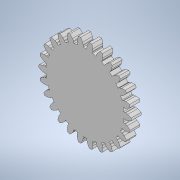
# Autodesk Inventor part: m1歯数26ギア3t
Saved by Autodesk Inventor 2020.2 (Build 242310000, 310)
## iProperties
Created: 2020-02-29
Part Number: m1歯数26ギア3t
Material: 一般
Document SubType Name: Modeling
Designer: aoyam
Density: 1 g/cm^3
Appearance: 既定
Author: aoyam
Autodesk Inventor part; units mm, degrees
ref_plane "YZ Plane" through (0, 0, 0) normal (1, 0, 0) x (0, 1, 0)
ref_plane "XZ Plane" through (0, 0, 0) normal (0, 1, 0) x (-1, 0, 0)
ref_plane "XY Plane" through (0, 0, 0) normal (0, 0, 1) x (1, 0, 0)
sketch "スケッチ1" plane through (0, 0, 0) normal (0, 0, 1) x (1, 0, 0)
  arc A0 (2.4708, 13.787) -> (2.4421, 13.6092) centre (3.6157, 13.511) ccw
  arc A1 (2.6541, 14.342) -> (2.4708, 13.787) centre (5.6233, 13.0538) ccw
  arc A2 (3.2141, 15.3428) -> (2.6541, 14.342) centre (7.7861, 12.1274) ccw
  arc A3 (1.3306, 13.6092) -> (1.3019, 13.787) centre (0.157, 13.511) ccw
  arc A4 (1.3019, 13.787) -> (1.1186, 14.342) centre (-1.8506, 13.0538) ccw
  arc A5 (1.1186, 14.342) -> (0.5586, 15.3428) centre (-4.0134, 12.1274) ccw
  arc A6 (2.4209, 13.1437) -> (1.3518, 13.1437) centre (1.8864, 1.4059) ccw
  arc A7 (0.5586, 15.3428) -> (-0.1598, 15.2555) centre (1.8864, 1.4059) ccw
  line L0 (2.4209, 13.1437) -> (2.4421, 13.6092)
  line L1 (1.3518, 13.1437) -> (1.3306, 13.6092)
  arc A8 (-0.5092, 13.5671) -> (-0.4945, 13.3876) centre (0.6685, 13.5731) ccw
  arc A9 (-1.6441, 13.2874) -> (-1.9549, 13.7824) centre (-4.5296, 11.821) ccw
  arc A10 (-0.1598, 15.2555) -> (-0.464, 14.1498) centre (5.0489, 13.2277) ccw
  arc A11 (-1.9549, 13.7824) -> (-2.7381, 14.6201) centre (-6.4078, 10.4039) ccw
  arc A12 (-2.7381, 14.6201) -> (-3.4148, 14.3634) centre (1.8864, 1.4059) ccw
  arc A13 (-1.5737, 13.1216) -> (-1.6441, 13.2874) centre (-2.6897, 12.7454) ccw
  line L2 (-1.4417, 12.6747) -> (-1.5737, 13.1216)
  arc A14 (-0.4037, 12.9306) -> (-1.4417, 12.6747) centre (1.8864, 1.4059) ccw
  line L3 (-0.4037, 12.9306) -> (-0.4945, 13.3876)
  arc A15 (-0.464, 14.1498) -> (-0.5092, 13.5671) centre (2.7272, 13.6096) ccw
  arc A16 (-3.3499, 12.6405) -> (-3.2927, 12.4697) centre (-2.2079, 12.9281) ccw
  arc A17 (-4.385, 12.0972) -> (-4.8051, 12.5035) centre (-6.8356, 9.9829) ccw
  arc A18 (-3.4148, 14.3634) -> (-3.4456, 13.217) centre (2.1278, 13.641) ccw
  arc A19 (-4.8051, 12.5035) -> (-5.7661, 13.1294) centre (-8.3201, 8.1575) ccw
  arc A20 (-5.7661, 13.1294) -> (-6.3617, 12.7182) centre (1.8864, 1.4059) ccw
  arc A21 (-4.2769, 11.9531) -> (-4.385, 12.0972) centre (-5.2705, 11.3208) ccw
  line L4 (-4.0418, 11.5508) -> (-4.2769, 11.9531)
  arc A22 (-3.0951, 12.0476) -> (-4.0418, 11.5508) centre (1.8864, 1.4059) ccw
  line L5 (-3.0951, 12.0476) -> (-3.2927, 12.4697)
  arc A23 (-3.4456, 13.217) -> (-3.3499, 12.6405) centre (-0.2178, 13.4562) ccw
  arc A24 (-5.8864, 11.0609) -> (-5.79, 10.9088) centre (-4.8464, 11.6135) ccw
  arc A25 (-6.7613, 10.2857) -> (-7.2665, 10.5796) centre (-8.6348, 7.6464) ccw
  arc A26 (-6.3617, 12.7182) -> (-6.1172, 11.5978) centre (-0.8073, 13.3433) ccw
  arc A27 (-7.2665, 10.5796) -> (-8.3493, 10.9574) centre (-9.6393, 5.5188) ccw
  arc A28 (-8.3493, 10.9574) -> (-8.8293, 10.4156) centre (1.8864, 1.4059) ccw
  arc A29 (-6.622, 10.1717) -> (-6.7613, 10.2857) centre (-7.4353, 9.3199) ccw
  line L6 (-6.2974, 9.8373) -> (-6.622, 10.1717)
  arc A30 (-5.4971, 10.5463) -> (-6.2974, 9.8373) centre (1.8864, 1.4059) ccw
  line L7 (-5.4971, 10.5463) -> (-5.79, 10.9088)
  arc A31 (-6.1172, 11.5978) -> (-5.8864, 11.0609) centre (-3.0405, 12.6025) ccw
  arc A32 (-7.9711, 8.9202) -> (-7.8411, 8.7956) centre (-7.0936, 9.7056) ccw
  arc A33 (-8.6351, 7.9582) -> (-9.196, 8.1226) centre (-9.8225, 4.9472) ccw
  arc A34 (-8.8293, 10.4156) -> (-8.3237, 9.3862) centre (-3.5858, 12.3518) ccw
  arc A35 (-9.196, 8.1226) -> (-10.3377, 8.2302) centre (-10.2887, 2.641) ccw
  arc A36 (-10.3377, 8.2302) -> (-10.6741, 7.5894) centre (1.8864, 1.4059) ccw
  arc A37 (-8.4725, 7.8808) -> (-8.6351, 7.9582) centre (-9.0584, 6.8591) ccw
  line L8 (-8.0774, 7.6338) -> (-8.4725, 7.8808)
  arc A38 (-7.47, 8.5137) -> (-8.0774, 7.6338) centre (1.8864, 1.4059) ccw
  line L9 (-7.47, 8.5137) -> (-7.8411, 8.7956)
  arc A39 (-8.3237, 9.3862) -> (-7.9711, 8.9202) centre (-5.5768, 11.0981) ccw
  arc A40 (-9.483, 6.3428) -> (-9.3269, 6.2529) centre (-8.8189, 7.3154) ccw
  arc A41 (-9.8975, 5.2498) -> (-10.4813, 5.2753) centre (-10.3298, 2.0422) ccw
  arc A42 (-10.6741, 7.5894) -> (-9.9369, 6.7109) centre (-6.0463, 10.7241) ccw
  arc A43 (-10.4813, 5.2753) -> (-11.6157, 5.1065) centre (-10.2305, -0.3086) ccw
  arc A44 (-11.6157, 5.1065) -> (-11.7889, 4.4038) centre (1.8864, 1.4059) ccw
  arc A45 (-9.7211, 5.2136) -> (-9.8975, 5.2498) centre (-10.0454, 4.0814) ccw
  line L10 (-9.2783, 5.0683) -> (-9.7211, 5.2136)
  arc A46 (-8.8991, 6.068) -> (-9.2783, 5.0683) centre (1.8864, 1.4059) ccw
  line L11 (-8.8991, 6.068) -> (-9.3269, 6.2529)
  arc A47 (-9.9369, 6.7109) -> (-9.483, 6.3428) centre (-7.6795, 9.0304) ccw
  arc A48 (-10.3341, 3.4785) -> (-10.161, 3.4286) centre (-9.9221, 4.5818) ccw
  arc A49 (-10.475, 2.3181) -> (-11.048, 2.203) centre (-10.1271, -0.8998) ccw
  arc A50 (-11.7889, 4.4038) -> (-10.8629, 3.7273) centre (-8.0458, 8.555) ccw
  arc A51 (-11.048, 2.203) -> (-12.109, 1.7677) centre (-9.4681, -3.1585) ccw
  arc A52 (-12.109, 1.7677) -> (-12.109, 1.044) centre (1.8864, 1.4059) ccw
  arc A53 (-10.295, 2.3251) -> (-10.475, 2.3181) centre (-10.339, 1.1482) ccw
  line L12 (-9.8303, 2.2901) -> (-10.295, 2.3251)
  arc A54 (-9.7015, 3.3514) -> (-9.8303, 2.2901) centre (1.8864, 1.4059) ccw
  line L13 (-9.7015, 3.3514) -> (-10.161, 3.4286)
  arc A55 (-10.8629, 3.7273) -> (-10.3341, 3.4785) centre (-9.2262, 6.5196) ccw
  arc A56 (-10.475, 0.4937) -> (-10.295, 0.4866) centre (-10.339, 1.6635) ccw
  arc A57 (-10.3341, -0.6667) -> (-10.8629, -0.9155) centre (-9.2262, -3.7078) ccw
  arc A58 (-12.109, 1.044) -> (-11.048, 0.6087) centre (-9.4681, 5.9703) ccw
  arc A59 (-10.8629, -0.9155) -> (-11.7889, -1.5921) centre (-8.0458, -5.7432) ccw
  arc A60 (-11.7889, -1.5921) -> (-11.6157, -2.2948) centre (1.8864, 1.4059) ccw
  arc A61 (-10.161, -0.6168) -> (-10.3341, -0.6667) centre (-9.9221, -1.77) ccw
  line L14 (-9.7015, -0.5396) -> (-10.161, -0.6168)
  arc A62 (-9.8303, 0.5217) -> (-9.7015, -0.5396) centre (1.8864, 1.4059) ccw
  line L15 (-9.8303, 0.5217) -> (-10.295, 0.4866)
  arc A63 (-11.048, 0.6087) -> (-10.475, 0.4937) centre (-10.1271, 3.7116) ccw
  arc A64 (-9.8975, -2.438) -> (-9.7211, -2.4018) centre (-10.0454, -1.2697) ccw
  arc A65 (-9.483, -3.531) -> (-9.9369, -3.8991) centre (-7.6795, -6.2186) ccw
  arc A66 (-11.6157, -2.2948) -> (-10.4813, -2.4635) centre (-10.2305, 3.1204) ccw
  arc A67 (-9.9369, -3.8991) -> (-10.6741, -4.7777) centre (-6.0463, -7.9124) ccw
  arc A68 (-10.6741, -4.7777) -> (-10.3377, -5.4185) centre (1.8864, 1.4059) ccw
  arc A69 (-9.3269, -3.4411) -> (-9.483, -3.531) centre (-8.8189, -4.5036) ccw
  line L16 (-8.8991, -3.2562) -> (-9.3269, -3.4411)
  arc A70 (-9.2783, -2.2566) -> (-8.8991, -3.2562) centre (1.8864, 1.4059) ccw
  line L17 (-9.2783, -2.2566) -> (-9.7211, -2.4018)
  arc A71 (-10.4813, -2.4635) -> (-9.8975, -2.438) centre (-10.3298, 0.7696) ccw
  arc A72 (-8.6351, -5.1464) -> (-8.4725, -5.069) centre (-9.0584, -4.0474) ccw
  arc A73 (-7.9711, -6.1084) -> (-8.3237, -6.5745) centre (-5.5768, -8.2863) ccw
  arc A74 (-10.3377, -5.4185) -> (-9.196, -5.3108) centre (-10.2887, 0.1708) ccw
  arc A75 (-8.3237, -6.5745) -> (-8.8293, -7.6039) centre (-3.5858, -9.54) ccw
  arc A76 (-8.8293, -7.6039) -> (-8.3493, -8.1456) centre (1.8864, 1.4059) ccw
  arc A77 (-7.8411, -5.9838) -> (-7.9711, -6.1084) centre (-7.0936, -6.8939) ccw
  line L18 (-7.47, -5.7019) -> (-7.8411, -5.9838)
  arc A78 (-8.0774, -4.822) -> (-7.47, -5.7019) centre (1.8864, 1.4059) ccw
  line L19 (-8.0774, -4.822) -> (-8.4725, -5.069)
  arc A79 (-9.196, -5.3108) -> (-8.6351, -5.1464) centre (-9.8225, -2.1354) ccw
  arc A80 (-6.7613, -7.474) -> (-6.622, -7.3599) centre (-7.4353, -6.5082) ccw
  arc A81 (-5.8864, -8.2491) -> (-6.1172, -8.786) centre (-3.0405, -9.7908) ccw
  arc A82 (-8.3493, -8.1456) -> (-7.2665, -7.7678) centre (-9.6393, -2.707) ccw
  arc A83 (-6.1172, -8.786) -> (-6.3617, -9.9065) centre (-0.8073, -10.5315) ccw
  arc A84 (-6.3617, -9.9065) -> (-5.7661, -10.3176) centre (1.8864, 1.4059) ccw
  arc A85 (-5.79, -8.097) -> (-5.8864, -8.2491) centre (-4.8464, -8.8017) ccw
  line L20 (-5.4971, -7.7345) -> (-5.79, -8.097)
  arc A86 (-6.2974, -7.0255) -> (-5.4971, -7.7345) centre (1.8864, 1.4059) ccw
  line L21 (-6.2974, -7.0255) -> (-6.622, -7.3599)
  arc A87 (-7.2665, -7.7678) -> (-6.7613, -7.474) centre (-8.6348, -4.8346) ccw
  arc A88 (-4.385, -9.2855) -> (-4.2769, -9.1414) centre (-5.2705, -8.509) ccw
  arc A89 (-3.3499, -9.8287) -> (-3.4456, -10.4052) centre (-0.2178, -10.6445) ccw
  arc A90 (-5.7661, -10.3176) -> (-4.8051, -9.6917) centre (-8.3201, -5.3458) ccw
  arc A91 (-3.4456, -10.4052) -> (-3.4148, -11.5517) centre (2.1278, -10.8293) ccw
  arc A92 (-3.4148, -11.5517) -> (-2.7381, -11.8083) centre (1.8864, 1.4059) ccw
  arc A93 (-3.2927, -9.6579) -> (-3.3499, -9.8287) centre (-2.2079, -10.1163) ccw
  line L22 (-3.0951, -9.2359) -> (-3.2927, -9.6579)
  arc A94 (-4.0418, -8.739) -> (-3.0951, -9.2359) centre (1.8864, 1.4059) ccw
  line L23 (-4.0418, -8.739) -> (-4.2769, -9.1414)
  arc A95 (-4.8051, -9.6917) -> (-4.385, -9.2855) centre (-6.8356, -7.1712) ccw
  arc A96 (-1.6441, -10.4756) -> (-1.5737, -10.3099) centre (-2.6897, -9.9336) ccw
  arc A97 (-0.5092, -10.7554) -> (-0.464, -11.338) centre (2.7272, -10.7979) ccw
  arc A98 (-2.7381, -11.8083) -> (-1.9549, -10.9706) centre (-6.4078, -7.5922) ccw
  arc A99 (-0.464, -11.338) -> (-0.1598, -12.4438) centre (5.0489, -10.416) ccw
  arc A100 (-0.1598, -12.4438) -> (0.5586, -12.531) centre (1.8864, 1.4059) ccw
  arc A101 (-0.4945, -10.5759) -> (-0.5092, -10.7554) centre (0.6685, -10.7614) ccw
  line L24 (-0.4037, -10.1188) -> (-0.4945, -10.5759)
  arc A102 (-1.4417, -9.8629) -> (-0.4037, -10.1188) centre (1.8864, 1.4059) ccw
  line L25 (-1.4417, -9.8629) -> (-1.5737, -10.3099)
  arc A103 (-1.9549, -10.9706) -> (-1.6441, -10.4756) centre (-4.5296, -9.0092) ccw
  arc A104 (1.3019, -10.9753) -> (1.3306, -10.7975) centre (0.157, -10.6992) ccw
  arc A105 (2.4708, -10.9753) -> (2.6541, -11.5302) centre (5.6233, -10.242) ccw
  arc A106 (0.5586, -12.531) -> (1.1186, -11.5302) centre (-4.0134, -9.3156) ccw
  arc A107 (2.6541, -11.5302) -> (3.2141, -12.531) centre (7.7861, -9.3156) ccw
  arc A108 (3.2141, -12.531) -> (3.9325, -12.4438) centre (1.8864, 1.4059) ccw
  arc A109 (2.4421, -10.7975) -> (2.4708, -10.9753) centre (3.6157, -10.6992) ccw
  line L26 (2.4209, -10.3319) -> (2.4421, -10.7975)
  arc A110 (1.3518, -10.3319) -> (2.4209, -10.3319) centre (1.8864, 1.4059) ccw
  line L27 (1.3518, -10.3319) -> (1.3306, -10.7975)
  arc A111 (1.1186, -11.5302) -> (1.3019, -10.9753) centre (-1.8506, -10.242) ccw
  arc A112 (4.2819, -10.7554) -> (4.2672, -10.5759) centre (3.1042, -10.7614) ccw
  arc A113 (5.4168, -10.4756) -> (5.7276, -10.9706) centre (8.3023, -9.0092) ccw
  arc A114 (3.9325, -12.4438) -> (4.2368, -11.338) centre (-1.2761, -10.416) ccw
  arc A115 (5.7276, -10.9706) -> (6.5108, -11.8083) centre (10.1805, -7.5922) ccw
  arc A116 (6.5108, -11.8083) -> (7.1875, -11.5517) centre (1.8864, 1.4059) ccw
  arc A117 (5.3464, -10.3099) -> (5.4168, -10.4756) centre (6.4624, -9.9336) ccw
  line L28 (5.2144, -9.8629) -> (5.3464, -10.3099)
  arc A118 (4.1764, -10.1188) -> (5.2144, -9.8629) centre (1.8864, 1.4059) ccw
  line L29 (4.1764, -10.1188) -> (4.2672, -10.5759)
  arc A119 (4.2368, -11.338) -> (4.2819, -10.7554) centre (1.0455, -10.7979) ccw
  arc A120 (7.1226, -9.8287) -> (7.0654, -9.6579) centre (5.9806, -10.1163) ccw
  arc A121 (8.1577, -9.2855) -> (8.5778, -9.6917) centre (10.6083, -7.1712) ccw
  arc A122 (7.1875, -11.5517) -> (7.2183, -10.4052) centre (1.6449, -10.8293) ccw
  arc A123 (8.5778, -9.6917) -> (9.5388, -10.3176) centre (12.0928, -5.3458) ccw
  arc A124 (9.5388, -10.3176) -> (10.1344, -9.9065) centre (1.8864, 1.4059) ccw
  arc A125 (8.0496, -9.1414) -> (8.1577, -9.2855) centre (9.0432, -8.509) ccw
  line L30 (7.8145, -8.739) -> (8.0496, -9.1414)
  arc A126 (6.8679, -9.2359) -> (7.8145, -8.739) centre (1.8864, 1.4059) ccw
  line L31 (6.8679, -9.2359) -> (7.0654, -9.6579)
  arc A127 (7.2183, -10.4052) -> (7.1226, -9.8287) centre (3.9905, -10.6445) ccw
  arc A128 (9.6591, -8.2491) -> (9.5627, -8.097) centre (8.6191, -8.8017) ccw
  arc A129 (10.5341, -7.474) -> (11.0392, -7.7678) centre (12.4075, -4.8346) ccw
  arc A130 (10.1344, -9.9065) -> (9.8899, -8.786) centre (4.58, -10.5315) ccw
  arc A131 (11.0392, -7.7678) -> (12.122, -8.1456) centre (13.412, -2.707) ccw
  arc A132 (12.122, -8.1456) -> (12.602, -7.6039) centre (1.8864, 1.4059) ccw
  arc A133 (10.3947, -7.3599) -> (10.5341, -7.474) centre (11.208, -6.5082) ccw
  line L32 (10.0701, -7.0255) -> (10.3947, -7.3599)
  arc A134 (9.2699, -7.7345) -> (10.0701, -7.0255) centre (1.8864, 1.4059) ccw
  line L33 (9.2699, -7.7345) -> (9.5627, -8.097)
  arc A135 (9.8899, -8.786) -> (9.6591, -8.2491) centre (6.8132, -9.7908) ccw
  arc A136 (11.7438, -6.1084) -> (11.6138, -5.9838) centre (10.8663, -6.8939) ccw
  arc A137 (12.4079, -5.1464) -> (12.9687, -5.3108) centre (13.5952, -2.1354) ccw
  arc A138 (12.602, -7.6039) -> (12.0964, -6.5745) centre (7.3585, -9.54) ccw
  arc A139 (12.9687, -5.3108) -> (14.1104, -5.4185) centre (14.0614, 0.1708) ccw
  arc A140 (14.1104, -5.4185) -> (14.4468, -4.7777) centre (1.8864, 1.4059) ccw
  arc A141 (12.2452, -5.069) -> (12.4079, -5.1464) centre (12.8311, -4.0474) ccw
  line L34 (11.8501, -4.822) -> (12.2452, -5.069)
  arc A142 (11.2427, -5.7019) -> (11.8501, -4.822) centre (1.8864, 1.4059) ccw
  line L35 (11.2427, -5.7019) -> (11.6138, -5.9838)
  arc A143 (12.0964, -6.5745) -> (11.7438, -6.1084) centre (9.3495, -8.2863) ccw
  arc A144 (13.2557, -3.531) -> (13.0996, -3.4411) centre (12.5916, -4.5036) ccw
  arc A145 (13.6702, -2.438) -> (14.2541, -2.4635) centre (14.1025, 0.7696) ccw
  arc A146 (14.4468, -4.7777) -> (13.7096, -3.8991) centre (9.819, -7.9124) ccw
  arc A147 (14.2541, -2.4635) -> (15.3884, -2.2948) centre (14.0032, 3.1204) ccw
  arc A148 (15.3884, -2.2948) -> (15.5616, -1.5921) centre (1.8864, 1.4059) ccw
  arc A149 (13.4938, -2.4018) -> (13.6702, -2.438) centre (13.8181, -1.2697) ccw
  line L36 (13.051, -2.2566) -> (13.4938, -2.4018)
  arc A150 (12.6719, -3.2562) -> (13.051, -2.2566) centre (1.8864, 1.4059) ccw
  line L37 (12.6719, -3.2562) -> (13.0996, -3.4411)
  arc A151 (13.7096, -3.8991) -> (13.2557, -3.531) centre (11.4522, -6.2186) ccw
  arc A152 (14.1068, -0.6667) -> (13.9337, -0.6168) centre (13.6948, -1.77) ccw
  arc A153 (14.2477, 0.4937) -> (14.8207, 0.6087) centre (13.8998, 3.7116) ccw
  arc A154 (15.5616, -1.5921) -> (14.6356, -0.9155) centre (11.8185, -5.7432) ccw
  arc A155 (14.8207, 0.6087) -> (15.8817, 1.044) centre (13.2408, 5.9703) ccw
  arc A156 (15.8817, 1.044) -> (15.8817, 1.7677) centre (1.8864, 1.4059) ccw
  arc A157 (14.0677, 0.4866) -> (14.2477, 0.4937) centre (14.1117, 1.6635) ccw
  line L38 (13.603, 0.5217) -> (14.0677, 0.4866)
  arc A158 (13.4742, -0.5396) -> (13.603, 0.5217) centre (1.8864, 1.4059) ccw
  line L39 (13.4742, -0.5396) -> (13.9337, -0.6168)
  arc A159 (14.6356, -0.9155) -> (14.1068, -0.6667) centre (12.9989, -3.7078) ccw
  arc A160 (14.2477, 2.3181) -> (14.0677, 2.3251) centre (14.1117, 1.1482) ccw
  arc A161 (14.1068, 3.4785) -> (14.6356, 3.7273) centre (12.9989, 6.5196) ccw
  arc A162 (15.8817, 1.7677) -> (14.8207, 2.203) centre (13.2408, -3.1585) ccw
  arc A163 (14.6356, 3.7273) -> (15.5616, 4.4038) centre (11.8185, 8.555) ccw
  arc A164 (15.5616, 4.4038) -> (15.3884, 5.1065) centre (1.8864, 1.4059) ccw
  arc A165 (13.9337, 3.4286) -> (14.1068, 3.4785) centre (13.6948, 4.5818) ccw
  line L40 (13.4742, 3.3514) -> (13.9337, 3.4286)
  arc A166 (13.603, 2.2901) -> (13.4742, 3.3514) centre (1.8864, 1.4059) ccw
  line L41 (13.603, 2.2901) -> (14.0677, 2.3251)
  arc A167 (14.8207, 2.203) -> (14.2477, 2.3181) centre (13.8998, -0.8998) ccw
  arc A168 (13.6702, 5.2498) -> (13.4938, 5.2136) centre (13.8181, 4.0814) ccw
  arc A169 (13.2557, 6.3428) -> (13.7096, 6.7109) centre (11.4522, 9.0304) ccw
  arc A170 (15.3884, 5.1065) -> (14.2541, 5.2753) centre (14.0032, -0.3086) ccw
  arc A171 (13.7096, 6.7109) -> (14.4468, 7.5894) centre (9.819, 10.7241) ccw
  arc A172 (14.4468, 7.5894) -> (14.1104, 8.2302) centre (1.8864, 1.4059) ccw
  arc A173 (13.0996, 6.2529) -> (13.2557, 6.3428) centre (12.5916, 7.3154) ccw
  line L42 (12.6719, 6.068) -> (13.0996, 6.2529)
  arc A174 (13.051, 5.0683) -> (12.6719, 6.068) centre (1.8864, 1.4059) ccw
  line L43 (13.051, 5.0683) -> (13.4938, 5.2136)
  arc A175 (14.2541, 5.2753) -> (13.6702, 5.2498) centre (14.1025, 2.0422) ccw
  arc A176 (12.4079, 7.9582) -> (12.2452, 7.8808) centre (12.8311, 6.8591) ccw
  arc A177 (11.7438, 8.9202) -> (12.0964, 9.3862) centre (9.3495, 11.0981) ccw
  arc A178 (14.1104, 8.2302) -> (12.9687, 8.1226) centre (14.0614, 2.641) ccw
  arc A179 (12.0964, 9.3862) -> (12.602, 10.4156) centre (7.3585, 12.3518) ccw
  arc A180 (12.602, 10.4156) -> (12.122, 10.9574) centre (1.8864, 1.4059) ccw
  arc A181 (11.6138, 8.7956) -> (11.7438, 8.9202) centre (10.8663, 9.7056) ccw
  line L44 (11.2427, 8.5137) -> (11.6138, 8.7956)
  arc A182 (11.8501, 7.6338) -> (11.2427, 8.5137) centre (1.8864, 1.4059) ccw
  line L45 (11.8501, 7.6338) -> (12.2452, 7.8808)
  arc A183 (12.9687, 8.1226) -> (12.4079, 7.9582) centre (13.5952, 4.9472) ccw
  arc A184 (10.5341, 10.2857) -> (10.3947, 10.1717) centre (11.208, 9.3199) ccw
  arc A185 (9.6591, 11.0609) -> (9.8899, 11.5978) centre (6.8132, 12.6025) ccw
  arc A186 (12.122, 10.9574) -> (11.0392, 10.5796) centre (13.412, 5.5188) ccw
  arc A187 (9.8899, 11.5978) -> (10.1344, 12.7182) centre (4.58, 13.3433) ccw
  arc A188 (10.1344, 12.7182) -> (9.5388, 13.1294) centre (1.8864, 1.4059) ccw
  arc A189 (9.5627, 10.9088) -> (9.6591, 11.0609) centre (8.6191, 11.6135) ccw
  line L46 (9.2699, 10.5463) -> (9.5627, 10.9088)
  arc A190 (10.0701, 9.8373) -> (9.2699, 10.5463) centre (1.8864, 1.4059) ccw
  line L47 (10.0701, 9.8373) -> (10.3947, 10.1717)
  arc A191 (11.0392, 10.5796) -> (10.5341, 10.2857) centre (12.4075, 7.6464) ccw
  arc A192 (8.1577, 12.0972) -> (8.0496, 11.9531) centre (9.0432, 11.3208) ccw
  arc A193 (7.1226, 12.6405) -> (7.2183, 13.217) centre (3.9905, 13.4562) ccw
  arc A194 (9.5388, 13.1294) -> (8.5778, 12.5035) centre (12.0928, 8.1575) ccw
  arc A195 (7.2183, 13.217) -> (7.1875, 14.3634) centre (1.6449, 13.641) ccw
  arc A196 (7.1875, 14.3634) -> (6.5108, 14.6201) centre (1.8864, 1.4059) ccw
  arc A197 (7.0654, 12.4697) -> (7.1226, 12.6405) centre (5.9806, 12.9281) ccw
  line L48 (6.8679, 12.0476) -> (7.0654, 12.4697)
  arc A198 (7.8145, 11.5508) -> (6.8679, 12.0476) centre (1.8864, 1.4059) ccw
  line L49 (7.8145, 11.5508) -> (8.0496, 11.9531)
  arc A199 (8.5778, 12.5035) -> (8.1577, 12.0972) centre (10.6083, 9.9829) ccw
  arc A200 (5.4168, 13.2874) -> (5.3464, 13.1216) centre (6.4624, 12.7454) ccw
  arc A201 (4.2819, 13.5671) -> (4.2368, 14.1498) centre (1.0455, 13.6096) ccw
  arc A202 (6.5108, 14.6201) -> (5.7276, 13.7824) centre (10.1805, 10.4039) ccw
  arc A203 (4.2368, 14.1498) -> (3.9325, 15.2555) centre (-1.2761, 13.2277) ccw
  arc A204 (3.9325, 15.2555) -> (3.2141, 15.3428) centre (1.8864, 1.4059) ccw
  arc A205 (4.2672, 13.3876) -> (4.2819, 13.5671) centre (3.1042, 13.5731) ccw
  line L50 (4.1764, 12.9306) -> (4.2672, 13.3876)
  arc A206 (5.2144, 12.6747) -> (4.1764, 12.9306) centre (1.8864, 1.4059) ccw
  line L51 (5.2144, 12.6747) -> (5.3464, 13.1216)
  arc A207 (5.7276, 13.7824) -> (5.4168, 13.2874) centre (8.3023, 11.821) ccw
  point P0 (0, 0)
  point P1 (13.051, 5.0683)
  point P2 (13.0996, 6.2529)
  point P3 (13.2557, 6.3428)
  point P4 (13.7096, 6.7109)
  point P5 (14.4468, 7.5894)
  point P6 (14.1104, 8.2302)
  point P7 (12.9687, 8.1226)
  point P8 (12.4079, 7.9582)
  point P9 (12.2452, 7.8808)
  point P10 (11.8501, 7.6338)
  point P11 (11.6138, 8.7956)
  point P12 (11.7438, 8.9202)
  point P13 (12.0964, 9.3862)
  point P14 (12.602, 10.4156)
  point P15 (12.122, 10.9574)
  point P16 (11.0392, 10.5796)
  point P17 (10.5341, 10.2857)
  point P18 (10.0701, 9.8373)
  point P19 (9.5627, 10.9088)
  point P20 (9.6591, 11.0609)
  point P21 (9.8899, 11.5978)
  point P22 (10.1344, 12.7182)
  point P23 (9.5388, 13.1294)
  point P24 (8.5778, 12.5035)
  point P25 (8.1577, 12.0972)
  point P26 (8.0496, 11.9531)
  point P27 (7.8145, 11.5508)
  point P28 (7.0654, 12.4697)
  point P29 (7.1226, 12.6405)
  point P30 (7.2183, 13.217)
  point P31 (7.1875, 14.3634)
  point P32 (6.5108, 14.6201)
  point P33 (5.7276, 13.7824)
  point P34 (5.4168, 13.2874)
  point P35 (5.3464, 13.1216)
  point P36 (5.2144, 12.6747)
  point P37 (4.2672, 13.3876)
  point P38 (4.2819, 13.5671)
  point P39 (4.2368, 14.1498)
  point P40 (3.9325, 15.2555)
  point P41 (3.2141, 15.3428)
  point P42 (2.6541, 14.342)
  point P43 (2.4708, 13.787)
  point P44 (2.4421, 13.6092)
  point P45 (1.3019, 13.787)
  point P46 (1.1186, 14.342)
  point P47 (0.5586, 15.3428)
  point P48 (-0.1598, 15.2555)
  point P49 (-0.464, 14.1498)
  point P50 (-0.5092, 13.5671)
  point P51 (-0.4945, 13.3876)
  point P52 (-0.4037, 12.9306)
  point P53 (-1.5737, 13.1216)
  point P54 (-1.6441, 13.2874)
  point P55 (-1.9549, 13.7824)
  point P56 (-2.7381, 14.6201)
  point P57 (-3.4148, 14.3634)
  point P58 (-3.4456, 13.217)
  point P59 (-3.3499, 12.6405)
  point P60 (-3.2927, 12.4697)
  point P61 (-4.0418, 11.5508)
  point P62 (-4.2769, 11.9531)
  point P63 (-4.385, 12.0972)
  point P64 (-4.8051, 12.5035)
  point P65 (-5.7661, 13.1294)
  point P66 (-6.3617, 12.7182)
  point P67 (-6.1172, 11.5978)
  point P68 (-5.8864, 11.0609)
  point P69 (-5.79, 10.9088)
  point P70 (-5.4971, 10.5463)
  point P71 (-6.2974, 9.8373)
  point P72 (-6.622, 10.1717)
  point P73 (-6.7613, 10.2857)
  point P74 (-7.2665, 10.5796)
  point P75 (-8.3493, 10.9574)
  point P76 (-8.8293, 10.4156)
  point P77 (-8.3237, 9.3862)
  point P78 (-7.9711, 8.9202)
  point P79 (-8.0774, 7.6338)
  point P80 (-8.4725, 7.8808)
  point P81 (-8.6351, 7.9582)
  point P82 (-9.196, 8.1226)
  point P83 (-10.3377, 8.2302)
  point P84 (-10.6741, 7.5894)
  point P85 (-9.9369, 6.7109)
  point P86 (-9.483, 6.3428)
  point P87 (-9.3269, 6.2529)
  point P88 (-8.8991, 6.068)
  point P89 (-9.8975, 5.2498)
  point P90 (-10.4813, 5.2753)
  point P91 (-11.6157, 5.1065)
  point P92 (-11.7889, 4.4038)
  point P93 (-10.8629, 3.7273)
  point P94 (-10.3341, 3.4785)
  point P95 (-10.161, 3.4286)
  point P96 (-9.7015, 3.3514)
  point P97 (-10.475, 2.3181)
  point P98 (-11.048, 2.203)
  point P99 (-12.109, 1.7677)
  point P100 (-12.109, 1.044)
  point P101 (-11.048, 0.6087)
  point P102 (-10.475, 0.4937)
  point P103 (-9.8303, 0.5217)
  point P104 (-9.7015, -0.5396)
  point P105 (-10.161, -0.6168)
  point P106 (-10.3341, -0.6667)
  point P107 (-10.8629, -0.9155)
  point P108 (-11.7889, -1.5921)
  point P109 (-11.6157, -2.2948)
  point P110 (-10.4813, -2.4635)
  point P111 (-9.8975, -2.438)
  point P112 (-9.483, -3.531)
  point P113 (-9.9369, -3.8991)
  point P114 (-10.6741, -4.7777)
  point P115 (-10.3377, -5.4185)
  point P116 (-9.196, -5.3108)
  point P117 (-8.6351, -5.1464)
  point P118 (-8.4725, -5.069)
  point P119 (-8.0774, -4.822)
  point P120 (-7.47, -5.7019)
  point P121 (-7.9711, -6.1084)
  point P122 (-8.3237, -6.5745)
  point P123 (-8.8293, -7.6039)
  point P124 (-8.3493, -8.1456)
  point P125 (-7.2665, -7.7678)
  point P126 (-6.7613, -7.474)
  point P127 (-6.2974, -7.0255)
  point P128 (-5.4971, -7.7345)
  point P129 (-5.79, -8.097)
  point P130 (-5.8864, -8.2491)
  point P131 (-6.1172, -8.786)
  point P132 (-6.3617, -9.9065)
  point P133 (-5.7661, -10.3176)
  point P134 (-4.8051, -9.6917)
  point P135 (-4.385, -9.2855)
  point P136 (-4.0418, -8.739)
  point P137 (-3.0951, -9.2359)
  point P138 (-3.3499, -9.8287)
  point P139 (-3.4456, -10.4052)
  point P140 (-3.4148, -11.5517)
  point P141 (-2.7381, -11.8083)
  point P142 (-1.9549, -10.9706)
  point P143 (-1.6441, -10.4756)
  point P144 (-1.4417, -9.8629)
  point P145 (-0.4945, -10.5759)
  point P146 (-0.5092, -10.7554)
  point P147 (-0.464, -11.338)
  point P148 (-0.1598, -12.4438)
  point P149 (0.5586, -12.531)
  point P150 (1.1186, -11.5302)
  point P151 (1.3019, -10.9753)
  point P152 (1.3306, -10.7975)
  point P153 (1.3518, -10.3319)
  point P154 (2.4421, -10.7975)
  point P155 (2.4708, -10.9753)
  point P156 (2.6541, -11.5302)
  point P157 (3.2141, -12.531)
  point P158 (3.9325, -12.4438)
  point P159 (4.2368, -11.338)
  point P160 (4.2819, -10.7554)
  point P161 (4.2672, -10.5759)
  point P162 (4.1764, -10.1188)
  point P163 (5.3464, -10.3099)
  point P164 (5.4168, -10.4756)
  point P165 (5.7276, -10.9706)
  point P166 (6.5108, -11.8083)
  point P167 (7.1875, -11.5517)
  point P168 (7.2183, -10.4052)
  point P169 (7.1226, -9.8287)
  point P170 (7.0654, -9.6579)
  point P171 (6.8679, -9.2359)
  point P172 (8.0496, -9.1414)
  point P173 (8.1577, -9.2855)
  point P174 (8.5778, -9.6917)
  point P175 (9.5388, -10.3176)
  point P176 (10.1344, -9.9065)
  point P177 (9.8899, -8.786)
  point P178 (9.6591, -8.2491)
  point P179 (10.0701, -7.0255)
  point P180 (10.5341, -7.474)
  point P181 (11.0392, -7.7678)
  point P182 (12.122, -8.1456)
  point P183 (12.602, -7.6039)
  point P184 (12.0964, -6.5745)
  point P185 (11.7438, -6.1084)
  point P186 (11.8501, -4.822)
  point P187 (12.4079, -5.1464)
  point P188 (12.9687, -5.3108)
  point P189 (14.1104, -5.4185)
  point P190 (14.4468, -4.7777)
  point P191 (13.7096, -3.8991)
  point P192 (13.2557, -3.531)
  point P193 (13.051, -2.2566)
  point P194 (13.6702, -2.438)
  point P195 (14.2541, -2.4635)
  point P196 (15.3884, -2.2948)
  point P197 (15.5616, -1.5921)
  point P198 (14.6356, -0.9155)
  point P199 (14.1068, -0.6667)
  dimension "d2" = 360
  constraints: 416 point on circle, 208 centre point, 104 end point, 2 coincident, 987 other
extrude "押し出し1" add sketch "スケッチ1" along normal blind 3
